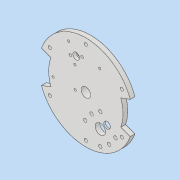
# Autodesk Inventor part: ThrustBearingMount
Saved by Autodesk Inventor 2017 (Build 210142000, 142)
## iProperties
Created: 2016-11-30
Part Number: ThrustBearingMount
Material: ABS Plastic
Document SubType Name: Modeling
Designer: techn
Density: 1.06 g/cm^3
Appearance: Smooth - White
Mass: 31.9611 g
Surface Area: 160.94 cm^2
Volume: 30.152 cm^3
Author: techn
Autodesk Inventor part; units mm, degrees
ref_plane "YZ Plane" through (0, 0, 0) normal (1, 0, 0) x (0, 1, 0)
ref_plane "XZ Plane" through (0, 0, 0) normal (0, 1, 0) x (-1, 0, 0)
ref_plane "XY Plane" through (0, 0, 0) normal (0, 0, 1) x (1, 0, 0)
sketch "Sketch5" plane through (0, 0, 0) normal (0, 0, 1) x (1, 0, 0)
  circle A0 centre (0, 0) radius 47.625
  dimension "d15" = 95.25
  constraints: 1 centre point, 1 coincident
  measures "d15" diameter of A0
extrude "Extrusion3" add sketch "Sketch5" along normal blind 4.7625
sketch "Sketch6" plane through (0, 0, 4.7625) normal (0, 0, 1) x (1, 0, 0)
  line L0 (0, 0) -> (0, 41.91)
  circle A0 centre (0, 41.91) radius 1.5875
  circle A1 centre (-36.2951, 20.955) radius 1.5875
  circle A2 centre (-36.2951, -20.955) radius 1.5875
  circle A3 centre (0, -41.91) radius 1.5875
  circle A4 centre (36.2951, -20.955) radius 1.5875
  circle A5 centre (36.2951, 20.955) radius 1.5875
  dimension "d18" = 41.91
  dimension "d19" = 3.175
  dimension "d22" = 360
  constraints: 6 centre point, 2 end point, 1 coincident, 1 vertical, 13 other
  measures "d18" distance of L0.start L0.end
  measures "d19" diameter of A0
extrude "Extrusion4" cut sketch "Sketch6" against normal blind 4.7625
sketch "Sketch7" plane through (0, 0, 0) normal (0, 0, -1) x (-1, 0, 0)
  circle A0 centre (0, 0) radius 11.303
  circle A1 centre (0, 0) radius 14.2875
  dimension "d26" = 22.606
  dimension "d27" = 28.575
  constraints: 2 centre point, 2 coincident
  measures "d26" diameter of A0
  measures "d27" diameter of A1
extrude "Extrusion5" add sketch "Sketch7" along normal blind 3.6068
sketch "Sketch9" plane through (0, 0, 0) normal (0, 0, -1) x (-1, 0, 0)
  circle A0 centre (0, 0) radius 4.7625
  dimension "d30" = 9.525
  constraints: 1 centre point, 1 coincident
  measures "d30" diameter of A0
extrude "Extrusion6" cut sketch "Sketch9" against normal through all
sketch "Sketch10" plane through (0, 0, 0) normal (0, 0, -1) x (-1, 0, 0)
  circle A0 centre (0, 0) radius 4.7625
  circle A1 centre (0, 0) radius 6.096
  dimension "d33" = 9.525
  dimension "d34" = 12.192
  constraints: 2 centre point, 2 coincident
  measures "d33" diameter of A0
  measures "d34" diameter of A1
extrude "Extrusion7" add sketch "Sketch10" along normal blind 3.6068
sketch "Sketch21" plane through (0, 0, 4.7625) normal (0, 0, 1) x (1, 0, 0)
  circle A0 centre (0, 0) radius 4.7625 projected
  line L0 (0, 0) -> (21.4033, -17.9595)
  line L1 (0, 0) -> (27.94, 0) construction
  circle A1 centre (21.4033, -17.9595) radius 3.302
  line L2 (21.4033, -17.9595) -> (14.5783, -24.7845)
  line L3 (21.4033, -17.9595) -> (31.0553, -17.9595) construction
  circle A2 centre (14.5783, -24.7845) radius 5.207
  circle A3 centre (14.5783, -24.7845) radius 18.034
  line L4 (14.5783, -24.7845) -> (14.5783, -9.5445)
  circle A4 centre (14.5783, -9.5445) radius 1.7145
  circle A5 centre (-0.6617, -24.7845) radius 1.7145
  circle A6 centre (14.5783, -40.0245) radius 1.7145
  circle A7 centre (29.8183, -24.7845) radius 1.7145
  dimension "d96" = 27.94
  dimension "d97" = 40
  dimension "d98" = 6.604
  dimension "d99" = 9.652
  dimension "d100" = 135
  dimension "d101" = 10.414
  dimension "d102" = 36.068
  dimension "d104" = 15.24
  dimension "d105" = 45
  dimension "d106" = 3.429
  dimension "d109" = 360
  constraints: 10 end point, 7 centre point, 4 coincident, 2 equal length, 2 horizontal, 9 other
  measures "d96" distance of L0.start L0.end
  measures "d97" angle of L0 L1
  measures "d98" diameter of A1
  measures "d99" distance of L2.start L2.end
  measures "d100" angle of L2 L3
  measures "d101" diameter of A2
  measures "d102" diameter of A3
  measures "d104" distance of L4.start L4.end
  measures "d105" angle of L2 L4
  measures "d106" diameter of A4
extrude "Extrusion19" cut sketch "Sketch21" against normal through all contours A1 L2 L0 | L0 L2 A1 | L4 L2 A2 | A2 L2 L4 | A4 | A5 | A6 | A7
sketch "Sketch22" plane through (0, 0, 0) normal (0, 0, -1) x (-1, 0, 0)
  circle A0 centre (-21.4033, -17.9595) radius 3.302 projected
  circle A1 centre (-21.4033, -17.9595) radius 6.35
  point P0 (0, 0)
  dimension "d113" = 12.7
  constraints: 1 centre point, 1 coincident
  measures "d113" diameter of A1
extrude "Extrusion20" cut sketch "Sketch22" against normal blind 3.175
sketch "Sketch23" plane through (0, 0, 4.7625) normal (0, 0, 1) x (1, 0, 0)
  circle A0 centre (14.5783, -24.7845) radius 5.207 projected
  line L0 (14.5783, -24.7845) -> (5.7395, -15.9456)
  line L1 (14.5783, -24.7845) -> (27.0783, -24.7845) construction
  line L2 (14.5783, -24.7845) -> (23.4171, -33.6233)
  circle A1 centre (5.7395, -15.9456) radius 1.7145
  circle A2 centre (23.4171, -33.6233) radius 1.7145
  point P0 (0, 0)
  dimension "d116" = 12.5
  dimension "d117" = 135
  dimension "d118" = 3.429
  dimension "d119" = 3.429
  constraints: 6 end point, 2 centre point, 2 coincident, 2 equal length, 1 collinear, 1 horizontal
  measures "d116" distance of L0.start L0.end
  measures "d117" angle of L1 L0
  measures "d118" diameter of A1
  measures "d119" diameter of A2
extrude "Extrusion21" cut sketch "Sketch23" against normal through all contours A1 | A2
sketch "Sketch24" plane through (0, 0, 4.7625) normal (0, 0, 1) x (1, 0, 0)
  circle A0 centre (0, 0) radius 4.7625 projected
  line L0 (0, 0) -> (-9.7732, 26.8517)
  line L1 (0, 0) -> (28.575, 0) construction
  circle A1 centre (-9.7732, 26.8517) radius 3.302
  circle A2 centre (-9.7732, 26.8517) radius 1.905
  line L2 (-9.7732, 26.8517) -> (-3.8062, 29.0235)
  line L3 (-9.7732, 26.8517) -> (-15.7403, 24.6799)
  circle A3 centre (-3.8062, 29.0235) radius 1.27
  circle A4 centre (-15.7403, 24.6799) radius 1.27
  dimension "d122" = 28.575
  dimension "d123" = 110
  dimension "d124" = 6.604
  dimension "d125" = 3.81
  dimension "d132" = 6.35
  dimension "d133" = 2.54
  dimension "d134" = 2.54
  constraints: 8 end point, 4 centre point, 4 coincident, 1 equal length, 1 horizontal, 1 perpendicular, 1 symmetric about line
  measures "d122" distance of L0.start L0.end
  measures "d123" angle of L1 L0
  measures "d124" diameter of A1
  measures "d125" diameter of A2
  measures "d132" distance of L2.start L2.end
  measures "d133" diameter of A3
  measures "d134" diameter of A4
extrude "Extrusion23" cut sketch "Sketch24" against normal blind 25.4 contours A2 L3 L0 | L0 L2 A2 | L3 A2 L2
extrude "Extrusion24" cut sketch "Sketch24" against normal blind 3.175 contours A1 L3 A2 L0 | L0 A2 L2 A1 | A1 L2 A2 L3
extrude "Extrusion25" cut sketch "Sketch24" against normal through all contours A3 | A4
sketch "Sketch26" plane through (0, 0, 4.7625) normal (0, 0, 1) x (1, 0, 0)
  circle A0 centre (-3.8062, 29.0235) radius 1.27 projected
  circle A1 centre (-9.7732, 26.8517) radius 3.302 projected
  line L0 (-3.8062, 29.0235) -> (-9.7732, 26.8517)
  line L1 (-9.7732, 26.8517) -> (-13.6174, 37.4134)
  line L2 (-9.7732, 26.8517) -> (-7.3191, 20.109)
  line L3 (-13.6174, 37.4134) -> (-17.3169, 36.0669)
  line L4 (-13.6174, 37.4134) -> (7.7447, 45.1885)
  line L5 (-7.3191, 20.109) -> (-11.0186, 18.7624)
  line L6 (-7.3191, 20.109) -> (14.043, 27.8841)
  circle A2 centre (-17.3169, 36.0669) radius 1.143
  circle A3 centre (7.7447, 45.1885) radius 1.143
  circle A4 centre (14.043, 27.8841) radius 1.143
  circle A5 centre (-11.0186, 18.7624) radius 1.143
  point P0 (0, 0)
  dimension "d137" = 11.2395
  dimension "d139" = 3.937
  dimension "d140" = 22.733
  dimension "d142" = 2.286
  dimension "d143" = 2.286
  dimension "d144" = 2.286
  dimension "d145" = 2.286
  dimension "d148" = 7.1755
  constraints: 14 end point, 5 perpendicular, 4 centre point, 4 coincident, 2 parallel, 1 collinear
  measures "d137" distance of L0.end L1.end
  measures "d139" distance of L1.end L3.end
  measures "d140" distance of L1.end L4.end
  measures "d142" diameter of A2
  measures "d143" diameter of A3
  measures "d144" diameter of A4
  measures "d145" diameter of A5
  measures "d148" distance of L0.end L2.end
extrude "Extrusion27" cut sketch "Sketch26" against normal through all contours A2 | A4 | A5
sketch "Sketch28" plane through (0, 0, 4.7625) normal (0, 0, 1) x (1, 0, 0)
  circle A0 centre (-33.02, -3.175) radius 1.143
  circle A1 centre (-10.795, -3.175) radius 1.143
  point P0 (0, 0)
  dimension "d164" = 2.286
  dimension "d165" = 2.286
  dimension "d166" = 22.225
  dimension "d170" = 3.175
  dimension "d171" = 10.795
  constraints: 2 centre point, 1 horizontal alignment
  measures "d164" diameter of A0
  measures "d165" diameter of A1
  measures "d166" distance of A1.centre A0.centre
  measures "d170" vertical distance of point (0, 0) A1.centre
  measures "d171" horizontal distance of point (0, 0) A1.centre
extrude "Extrusion28" cut sketch "Sketch28" against normal up to surface (4.7625 mm away)
sketch "Sketch29" plane through (0, 0, 4.7625) normal (0, 0, 1) x (1, 0, 0)
  circle A0 centre (0, 0) radius 47.625 projected
  circle A1 centre (0, 0) radius 37.465
  line L0 (0, 0) -> (-44.7529, 16.2887)
  line L1 (0, 0) -> (47.625, 0) construction
  line L2 (0, 0) -> (-44.7529, -16.2887)
  line L3 (0, 0) -> (47.625, 0) construction
  line L4 (0, 0) -> (44.7529, 16.2887)
  line L5 (0, 0) -> (47.625, 0) construction
  line L6 (0, 0) -> (44.7529, -16.2887)
  line L7 (0, 0) -> (47.625, 0) construction
  arc A2 (-35.2056, 12.8138) -> (-35.2056, -12.8138) centre (0, 0) ccw
  arc A3 (35.2056, -12.8138) -> (35.2056, 12.8138) centre (0, 0) ccw
  dimension "d172" = 10.16
  dimension "d173" = 160
  dimension "d174" = 160
  dimension "d175" = 20
  dimension "d176" = 20
  constraints: 16 end point, 12 point on circle, 4 equal length, 4 horizontal, 4 point on line, 3 centre point, 1 concentric
  measures "d172" radial gap between concentric circles of A0 A1
  measures "d173" angle of L1 L0
  measures "d174" angle of L2 L3
  measures "d175" angle of L5 L4
  measures "d176" angle of L6 L7
extrude "Extrusion29" cut sketch "Sketch29" against normal blind 25.4 contours A0 L6 A1 L4 | L0 A1 L2 A0
body "Solid2"
